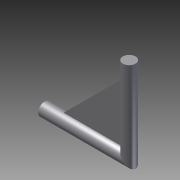
# Autodesk Inventor part: corner_prop
Saved by Autodesk Inventor 2011 (Build 150239000, 239)
## iProperties
Created: 2013-01-17
Part Number: corner_prop
Document SubType Name: Modeling
Designer: Christopher
Density: 1 g/cm^3
Author: Christopher
Autodesk Inventor part; units mm, degrees
ref_plane "YZ Plane" through (0, 0, 0) normal (1, 0, 0) x (0, 1, 0)
ref_plane "XZ Plane" through (0, 0, 0) normal (0, 1, 0) x (-1, 0, 0)
sketch "Sketch1" plane through (0, 0, 0) normal (0, 0, 1) x (1, 0, 0)
  line L0 (-254, 0) -> (0, 0)
  line L1 (0, 0) -> (0, 254)
  line L2 (-215.5261, 0) -> (0, 215.5261)
  dimension "d0" = 254
  dimension "d1" = 254
  dimension "d2" = 90
  dimension "d5" = 152.4
  dimension "d6" = 45
  constraints: 6 end point, 2 point on line, 1 horizontal
  measures "d0" distance of L0.start L0.end
  measures "d1" distance of L0.end L1.end
  measures "d2" angle of L0 L1
  measures "d5" distance from line of L2 L0.end
  measures "d6" angle of L1 L2
ref_plane "Work Plane1" through (-254, 0, 0) normal (1, 0, 0) x (0, 1, 0)
sketch "Sketch2" plane through (-254, 0, 0) normal (1, 0, 0) x (0, 1, 0)
  circle A0 centre (0, 0) radius 19.05
  dimension "d3" = 38.1
  constraints: 1 centre point, 1 coincident
  measures "d3" diameter of A0
sweep "Sweep1" add profiles "Sketch2" path "Sketch1" path curves L0 L1
extrude "Extrusion1" add sketch "Sketch1" against normal blind 3.175
body "Solid1"
